Ring v4 (Autodesk Fusion 360 design; units mm, degrees)
Autodesk Fusion 360 part; units mm, degrees
sketch "Sketch1" plane through (0, 0, 0) normal (0, 1, 0) x (1, 0, 0)
  circle A0 centre (0, 0) radius 25.4 construction
  circle A1 centre (0, 0) radius 24.65
  circle A2 centre (0, 0) radius 20.65
  dimension "d6" = -0.75
  dimension "d7" = 50.8
  dimension "d8" = -4.75
  constraint coincident A0.centre A1.centre
  measures "d7" diameter of A0
extrude "Extrude1" add sketch "Sketch1" along normal mid plane 10
equation "cardboard_offset = -0.75 mm"
equation "d6 = cardboard_offset"
equation "d8 = cardboard_offset - 4 mm"
